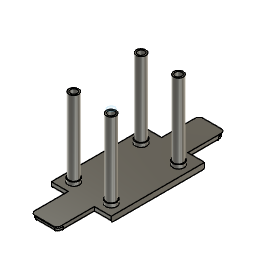
Micromouse_Gesamtaufbau_v8 (Autodesk Fusion 360 archive; units mm, degrees)
design "Mouse_Layout_MotorMount"
Autodesk Fusion 360 part; units mm, degrees
sketch "Skizze1" plane through (0, 0, 0) normal (0, 0, 1) x (1, 0, 0)
  line L0 (45, -30) -> (45, -50)
  line L1 (45, -50) -> (-45, -50)
  line L2 (-45, -50) -> (-45, -30)
  arc A0 (45, 0) -> (-45, 0) centre (0, 0) ccw
  line L3 (-45, 0) -> (-36, 0)
  line L4 (-36, 0) -> (-36, -30)
  line L5 (-36, -30) -> (-45, -30)
  line L6 (36, 0) -> (36, -30)
  line L7 (36, -30) -> (45, -30)
  line L8 (36, 0) -> (45, 0)
  dimension "d1" = 90
  dimension "d2" = 50
  dimension "d3" = 9
  dimension "d4" = 30
  dimension "d5" = 9
  dimension "d6" = 30
  constraint coincident A0.centre origin
  constraint vertical L0
  constraint horizontal L1
  constraint vertical L2
  constraint horizontal L3
  constraint vertical L4
  constraint horizontal L5
  constraint vertical L6
  constraint horizontal L7
  measures "d1" diameter of A0
  measures "d2" distance of A0.end L1.end
  measures "d3" distance of A0.end L3.end
  measures "d4" distance of A0.end L2.end
  measures "d5" distance of A0.start L6.start
  measures "d6" distance of A0.start L0.start
extrude "Extrusion1" add sketch "Skizze1" along normal blind 1.6 makes body 1
sketch "Skizze2" plane through (0, 0, 1.6) normal (0, 0, 1) x (-1, 0, 0)
  line L0 (-36, 30) -> (-36, 0)
  line L1 (-36, 0) -> (-45, 0)
  arc A0 (-45, 0) -> (45, 0) centre (0, 0) ccw
  line L2 (45, 0) -> (36, 0)
  line L3 (36, 0) -> (36, 30)
  line L4 (36, 30) -> (45, 30)
  line L5 (45, 30) -> (45, 50)
  line L6 (45, 50) -> (-45, 50)
  line L7 (-45, 50) -> (-45, 30)
  line L8 (-45, 30) -> (-36, 30)
  line L9 (36, 15) -> (36, 24)
  line L10 (36, 15) -> (36, 6)
  circle A1 centre (26, 24) radius 1.5
  circle A2 centre (16, 24) radius 1.5
  circle A3 centre (26, 6) radius 1.5
  circle A4 centre (16, 6) radius 1.5
  line L11 (36, 15) -> (36, 9)
  line L12 (36, 9) -> (11, 9)
  line L13 (11, 9) -> (11, 21)
  line L14 (11, 21) -> (36, 21)
  line L15 (36, 21) -> (36, 9)
  line L16 (36, 24) -> (36, 27)
  line L17 (36, 27) -> (4, 27)
  line L18 (4, 27) -> (4, 2)
  line L19 (4, 2) -> (36, 2)
  line L20 (36, 2) -> (36, 27)
  line L21 (-36, 27) -> (-4, 27)
  line L22 (-4, 27) -> (-4, 2)
  line L23 (-4, 2) -> (-36, 2)
  line L24 (-36, 2) -> (-36, 27)
  line L25 (-11, 21) -> (-36, 21)
  line L26 (-36, 21) -> (-11, 21)
  line L27 (-11, 21) -> (-11, 9)
  line L28 (-11, 9) -> (-36, 9)
  line L29 (-36, 9) -> (-36, 21)
  circle A5 centre (-16, 6) radius 1.5
  circle A6 centre (-26, 6) radius 1.5
  circle A7 centre (-16, 24) radius 1.5
  circle A8 centre (-26, 24) radius 1.5
  dimension "d10" = 9
  dimension "d11" = 9
  dimension "d12" = 10
  dimension "d13" = 10
  dimension "d14" = 10
  dimension "d15" = 10
  dimension "d16" = 3
  dimension "d17" = 3
  dimension "d18" = 3
  dimension "d19" = 3
  dimension "d20" = 6
  dimension "d21" = 25
  dimension "d22" = 12
  dimension "d23" = 3
  dimension "d24" = 32
  dimension "d25" = 25
  dimension "d30" = 32
  dimension "d31" = 25
  dimension "d32" = 25
  dimension "d33" = 12
  dimension "d35" = 10
  dimension "d37" = 10
  dimension "d38" = 3
  dimension "d39" = 3
  dimension "d40" = 3
  dimension "d41" = 3
  dimension "d42" = 10
  dimension "d43" = 10
  constraint midpoint L3 L9.start
  constraint horizontal L12
  constraint vertical L13
  constraint horizontal L14
  constraint vertical L15
  constraint coincident L3 L16.end
  constraint parallel L3 L16
  constraint horizontal L17
  constraint vertical L18
  constraint horizontal L19
  constraint vertical L20
  constraint coincident L0 L21.start
  constraint horizontal L21
  constraint vertical L22
  constraint horizontal L23
  constraint vertical L24
  constraint perpendicular L22 L25
  constraint horizontal L26
  constraint vertical L27
  constraint horizontal L28
  constraint vertical L29
  measures "d10" distance of L9.start L9.end
  measures "d11" distance of L9.start L10.end
  measures "d12" distance of L10.end A3.centre
  measures "d13" distance of A3.centre A4.centre
  measures "d14" distance of L9.end A1.centre
  measures "d15" distance of A1.centre A2.centre
  measures "d16" diameter of A1
  measures "d17" diameter of A2
  measures "d18" diameter of A3
  measures "d19" diameter of A4
  measures "d20" distance of L9.start L11.end
  measures "d21" distance of L11.end L12.end
  measures "d22" distance of L11.end L14.end
  measures "d23" distance of L9.end L16.end
  measures "d24" distance of L16.end L17.end
  measures "d25" distance of L16.end L19.end
  measures "d30" distance of L21.start L21.end
  measures "d31" distance of L21.start L23.end
  measures "d32" distance of L25.end L25.start
  measures "d33" distance of L25.end L28.end
  measures "d35" distance of A5.centre A6.centre
  measures "d37" distance of A7.centre A8.centre
  measures "d38" diameter of A5
  measures "d39" diameter of A6
  measures "d40" diameter of A7
  measures "d41" diameter of A8
  measures "d42" distance of L24 A6.centre
  measures "d43" distance of L24 A8.centre
extrude "Extrusion2" cut sketch "Skizze2" against normal blind 1.6 contours A1 | A2 | A3 | A4 bodies 1
mirror "Spiegeln1" about plane through (0, 0, 0) normal (1, 0, 0) of "Extrusion2"
extrude "Extrusion3" cut sketch "Skizze2" against normal blind 2 contours L0 L1 A0 L2 L3 L4 L5 L6 L7 L8 L17 L18 L19 L21 L22 L23 bodies 1 makes body 2 at (7.5869, -11.9483, 0)
extrude "Extrusion4" cut sketch "Skizze2" against normal blind 2 contours L0 L1 A0 L2 L3 L4 L5 L6 L7 L8 L17 L18 L19 L21 L22 L23 bodies 2 1
extrude "Extrusion5" cut sketch "Skizze2" against normal blind 2 contours L0 L21 L22 L23 L24 L25 L26 L27 L28 | L0 L24 L25 L26 L27 L28 L29 bodies 2
sketch "Skizze3" plane through (0, 0, 0) normal (0, 0, -1) x (1, 0, 0)
  line L0 (-36, 2) -> (-4, 2)
  line L1 (-4, 2) -> (-4, 27)
  line L2 (-4, 27) -> (-36, 27)
  line L3 (-36, 27) -> (-36, 2)
  circle A0 centre (-26, 24) radius 1.5
  circle A1 centre (-26, 6) radius 1.5
  circle A2 centre (-16, 24) radius 1.5
  circle A3 centre (-16, 6) radius 1.5
  line L4 (-29, 27) -> (-13, 27)
  line L5 (-13, 27) -> (-13, 2)
  line L6 (-13, 2) -> (-29, 2)
  line L7 (-29, 2) -> (-29, 27)
  circle A4 centre (-26, 24) radius 1.5
  circle A5 centre (-16, 24) radius 1.5
  circle A6 centre (-16, 6) radius 1.5
  circle A7 centre (-26, 6) radius 1.5
  constraint horizontal L4
  constraint vertical L5
  constraint horizontal L6
  constraint vertical L7
  constraint coincident L0 L5.end
  constraint coincident L2 L4.start
  constraint concentric A0 A4
  constraint concentric A2 A5
  constraint concentric A3 A6
  constraint concentric A1 A7
extrude "Extrusion6" add sketch "Skizze3" along normal blind 1.9 contours L0 L2 L4 L5 L6 L7 | A0 A4 | A1 A7 | A2 A5 | A3 A6 bodies 1 2
extrude "Extrusion7" cut sketch "Skizze2" against normal blind 1.6 contours L3 L9 L10 L12 L13 L14 L16 L17 L18 L19 L20 | L3 L9 L10 L11 L12 L13 L14 L15 L20 bodies 1
extrude "Extrusion8" add sketch "Skizze3" against normal blind 21.9 contours A0 A4 | A1 A7 | A2 A5 | A3 A6 bodies 1
sketch "Skizze4" plane through (0, -27, 0) normal (0, -1, 0) x (1, 0, 0)
  line L0 (-13, 0) -> (-29, 0)
  line L1 (-29, 0) -> (-29, -1.9)
  line L2 (-29, -1.9) -> (-13, -1.9)
  line L3 (-13, -1.9) -> (-13, 0)
  line L4 (-24.5, 0) -> (-17.5, 0)
  line L5 (-17.5, 0) -> (-17.5, -1.9)
  line L6 (-17.5, -1.9) -> (-24.5, -1.9)
  line L7 (-24.5, -1.9) -> (-24.5, 0)
  dimension "d56" = 7
  constraint horizontal L4
  constraint vertical L5
  constraint horizontal L6
  constraint vertical L7
  constraint coincident L2 L5.end
  constraint coincident L0 L4.start
  measures "d56" distance of L4.start L4.end
extrude "Extrusion9" add sketch "Skizze4" along normal blind 10 contours L0 L2 L4 L5 L6 L7 bodies 1
sketch "Skizze5" plane through (0, -2, 0) normal (0, 1, 0) x (-1, 0, 0)
  line L0 (29, 0) -> (13, 0)
  line L1 (13, 0) -> (13, -1.9)
  line L2 (13, -1.9) -> (29, -1.9)
  line L3 (29, -1.9) -> (29, 0)
  line L4 (17.5, 0) -> (24.5, 0)
  line L5 (24.5, 0) -> (24.5, -1.9)
  line L6 (24.5, -1.9) -> (17.5, -1.9)
  line L7 (17.5, -1.9) -> (17.5, 0)
  constraint horizontal L4
  constraint vertical L5
  constraint horizontal L6
  constraint vertical L7
  constraint coincident L2 L5.end
  constraint coincident L0 L4.start
extrude "Extrusion10" add sketch "Skizze5" along normal blind 10 contours L0 L2 L4 L5 L6 L7 bodies 1
fillet "Abrundung1" radius 3.5 2 edges at (-21, -37, -1.9) (-21, 8, -1.9) on bodies 1
fillet "Abrundung2" radius 1 14 edges at (-24.5, 1.4436, -1.9) (-24.5, 6.7106, -1.3875) (-17.5, 1.4436, -1.9) (-17.5, 6.7106, -1.3875) (-13, -14.5, -1.9) (-26.75, -2, -1.9) (-15.25, -2, -1.9) (-15.25, -27, -1.9) (-17.5, -30.4436, -1.9) (-17.5, -35.7106, -1.3875) (-24.5, -30.4436, -1.9) (-24.5, -35.7106, -1.3875) (-26.75, -27, -1.9) (-29, -14.5, -1.9) on bodies 1
sketch "Skizze6" plane through (0, 0, 21.9) normal (0, 0, 1) x (-1, 0, 0)
  circle A0 centre (26, 6) radius 1.5
  circle A1 centre (26, 6) radius 0.9
  circle A2 centre (16, 6) radius 0.9
  circle A3 centre (26, 24) radius 0.9
  circle A4 centre (16, 24) radius 0.9
  dimension "d65" = 1.8
  dimension "d66" = 1.8
  dimension "d67" = 1.8
  dimension "d68" = 1.8
  constraint concentric A0 A1
  measures "d65" diameter of A1
  measures "d66" diameter of A2
  measures "d67" diameter of A3
  measures "d68" diameter of A4
extrude "Extrusion11" cut sketch "Skizze6" against normal blind 12 contours A1 | A2 | A3 | A4 bodies 1
fillet "Abrundung3" radius 0.5 4 edges at (-27.3985, -6.5424, 21.9) (-17.3985, -6.5424, 21.9) (-17.3985, -24.5424, 21.9) (-27.3985, -24.5424, 21.9) on bodies 1
sketch "Skizze7" plane through (0, 0, 21.9) normal (0, 0, 1) x (-1, 0, 0)
  circle A0 centre (16, 24) radius 0.9
  circle A1 centre (16, 24) radius 1
  circle A2 centre (26, 6) radius 1.3
  circle A3 centre (16, 6) radius 1.3
  circle A4 centre (26, 24) radius 1.3
  circle A5 centre (16, 24) radius 1.3
  circle A6 centre (26, 6) radius 1.5
  circle A7 centre (16, 6) radius 1.5
  circle A8 centre (26, 24) radius 1.5
  circle A9 centre (16, 24) radius 1.5
  dimension "d73" = 2.6
  dimension "d74" = 2.6
  dimension "d75" = 2.6
  dimension "d76" = 3
  dimension "d77" = 3
  dimension "d78" = 3
  dimension "d79" = 3
  dimension "d82" = 2.6
  constraint concentric A0 A5
  constraint concentric A2 A6
  constraint concentric A3 A7
  constraint concentric A4 A8
  constraint concentric A5 A9
  measures "d73" diameter of A3
  measures "d74" diameter of A4
  measures "d75" diameter of A5
  measures "d76" diameter of A6
  measures "d77" diameter of A7
  measures "d78" diameter of A8
  measures "d79" diameter of A9
  measures "d82" diameter of A2
extrude "Extrusion12" cut sketch "Skizze7" against normal blind 21.9 contours A6 | A7 | A8 | A9 bodies 1
sketch "Skizze8" plane through (0, 0, -1.9) normal (0, 0, -1) x (1, 0, 0)
  line L0 (-18.5, 26) -> (-18.5, 33.8871)
  line L1 (-18.5, 33.8871) -> (-23.5, 33.8871)
  line L2 (-23.5, 33.8871) -> (-23.5, 26)
  line L3 (-23.5, 26) -> (-28, 26)
  line L4 (-28, 26) -> (-28, 3)
  line L5 (-28, 3) -> (-23.5, 3)
  line L6 (-23.5, 3) -> (-23.5, -4.8871)
  line L7 (-23.5, -4.8871) -> (-18.5, -4.8871)
  line L8 (-18.5, -4.8871) -> (-18.5, 3)
  line L9 (-18.5, 3) -> (-14, 3)
  line L10 (-14, 3) -> (-14, 26)
  line L11 (-14, 26) -> (-18.5, 26)
  line L12 (-13, 27) -> (-13, 2)
  line L13 (-29, 2) -> (-29, 27)
  line L14 (-13, 27) -> (-13, 37)
  line L15 (-13, 37) -> (-29, 37)
  line L16 (-29, 37) -> (-29, 27)
  line L17 (-13, 2) -> (-13, -8)
  line L18 (-13, -8) -> (-29, -8)
  line L19 (-29, -8) -> (-29, 2)
  constraint vertical L12
  constraint vertical L13
  constraint vertical L14
  constraint horizontal L15
  constraint vertical L16
  constraint vertical L17
  constraint horizontal L18
  constraint vertical L19
extrude "Extrusion13" cut sketch "Skizze8" against normal blind 1.4 contours L0 L1 L2 L3 L4 L5 L6 L7 L8 L9 L10 L11 | L12 L13 L14 L15 L16 L17 L18 L19 bodies 1
sketch "Skizze9" plane through (0, 0, 0) normal (0, 0, 1) x (-1, 0, 0)
  circle A0 centre (16, 6) radius 1.3
  circle A1 centre (26, 24) radius 1.3
  circle A2 centre (26, 6) radius 1.3
  circle A3 centre (16, 24) radius 1.3
  spline S0 degree 3 poles (17.5, 35.8081) (17.5, 35.9658) (17.5285, 36.153) (17.627, 36.4268) (17.7057, 36.566) (17.8787, 36.7656) (18.0032, 36.8615) (18.2336, 36.9678) (18.3773, 37) (18.5, 37) knots 1.603619 1.603619 1.603619 1.603619 1.650953 1.650953 1.690911 1.690911 1.730212 1.730212 1.767024 1.767024 1.767024 1.767024
  line L0 (17.5, 35.8081) -> (17.5, 27)
  line L1 (17.5, 27) -> (13, 27)
  line L2 (13, 27) -> (13, 2)
  line L3 (13, 2) -> (17.5, 2)
  line L4 (17.5, 2) -> (17.5, -6.8081)
  spline S1 degree 3 poles (18.5, -8) (18.3827, -8) (18.245, -7.9706) (18.0235, -7.8732) (17.9025, -7.7854) (17.7235, -7.593) (17.6383, -7.4507) (17.531, -7.1676) (17.5, -6.9726) (17.5, -6.8081) knots 1.060205 1.060205 1.060205 1.060205 1.095405 1.095405 1.132785 1.132785 1.174245 1.174245 1.223607 1.223607 1.223607 1.223607
  line L5 (18.5, -8) -> (23.5, -8)
  spline S2 degree 3 poles (24.5, -6.8081) (24.5, -6.9726) (24.469, -7.1676) (24.3617, -7.4507) (24.2765, -7.593) (24.0975, -7.7854) (23.9765, -7.8732) (23.755, -7.9706) (23.6173, -8) (23.5, -8) knots 1.603606 1.603606 1.603606 1.603606 1.652968 1.652968 1.694428 1.694428 1.731808 1.731808 1.767008 1.767008 1.767008 1.767008
  line L6 (24.5, -6.8081) -> (24.5, 2)
  line L7 (24.5, 2) -> (29, 2)
  line L8 (29, 2) -> (29, 27)
  line L9 (29, 27) -> (24.5, 27)
  line L10 (24.5, 27) -> (24.5, 35.8081)
  spline S3 degree 3 poles (23.5, 37) (23.6227, 37) (23.7664, 36.9678) (23.9968, 36.8615) (24.1213, 36.7656) (24.2943, 36.566) (24.373, 36.4268) (24.4715, 36.153) (24.5, 35.9658) (24.5, 35.8081) knots 1.060215 1.060215 1.060215 1.060215 1.097027 1.097027 1.136328 1.136328 1.176286 1.176286 1.22362 1.22362 1.22362 1.22362
  line L11 (23.5, 37) -> (18.5, 37)
  circle A4 centre (16, 6) radius 1.3
  circle A5 centre (16, 6) radius 1.5
  circle A6 centre (26, 6) radius 1.3
  circle A7 centre (26, 6) radius 1.5
  circle A8 centre (16, 24) radius 1.3
  circle A9 centre (16, 24) radius 1.5
  circle A10 centre (26, 24) radius 1.3
  circle A11 centre (26, 24) radius 1.5
  constraint concentric A0 A4
  constraint concentric A4 A5
  constraint concentric A2 A6
  constraint concentric A2 A7
  constraint concentric A3 A8
  constraint concentric A8 A9
  constraint concentric A1 A10
  constraint concentric A10 A11
extrude "Extrusion14" add sketch "Skizze9" along normal blind 1 contours A5 | A7 | A9 | A11 bodies 1
extrude "Extrusion15" add 1 faces at (-22.1667, -18.6667, -0.5) along direction (0, 0, -1) blind 1 on bodies 1 bodies 1
sketch "Skizze10" plane through (0, 0, 21.9) normal (0, 0, 1) x (-1, 0, 0)
  circle A0 centre (16, 24) radius 0.9
  circle A1 centre (16, 24) radius 1
sketch "Skizze11" plane through (0, 0, 0) normal (1, 0, 0) x (0, 1, 0)
  line L0 (-25, 21.9) -> (-25.5, 21.9)
  line L1 (-25.5, 21.9) -> (-25.5, 20.9)
  line L2 (-25.5, 20.9) -> (-4, 20.9)
  line L3 (-4, 20.9) -> (-4, 21.9)
  line L4 (-4, 21.9) -> (-25, 21.9)
  constraint horizontal L0
  constraint perpendicular L0 L1
  constraint perpendicular L1 L2
  constraint perpendicular L2 L3
  constraint perpendicular L1 L4
extrude "Extrusion16" cut sketch "Skizze11" against normal blind 32 bodies 1
fillet "Abrundung5" radius 0.5 14 edges at (-17.5, -31.1218, -1.5) (-17.7132, -36.1881, -1.5) (-21, -36.6871, -1.5) (-24.2868, -36.1881, -1.5) (-24.5, -31.1218, -1.5) (-24.5, 2.1218, -1.5) (-24.2859, 7.1906, -1.5) (-21, 7.6871, -1.5) (-17.7141, 7.1906, -1.5) (-17.5, 2.1218, -1.5) (-15.25, -27, -1.5) (-26.75, -27, -1.5) (-26.75, -2, -1.5) (-15.25, -2, -1.5) on bodies 1

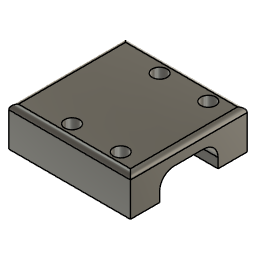
design "Mouse_Motor_Clamp_Upper"
Autodesk Fusion 360 part; units mm, degrees
sketch "Skizze1" plane through (0, 0, 0) normal (0, 0, 1) x (1, 0, 0)
  line L0 (45, -30) -> (45, -50)
  line L1 (45, -50) -> (-45, -50)
  line L2 (-45, -50) -> (-45, -30)
  arc A0 (45, 0) -> (-45, 0) centre (0, 0) ccw
  line L3 (-45, 0) -> (-36, 0)
  line L4 (-36, 0) -> (-36, -30)
  line L5 (-36, -30) -> (-45, -30)
  line L6 (36, 0) -> (36, -30)
  line L7 (36, -30) -> (45, -30)
  line L8 (36, 0) -> (45, 0)
  dimension "d1" = 90
  dimension "d2" = 50
  dimension "d3" = 9
  dimension "d4" = 30
  dimension "d5" = 9
  dimension "d6" = 30
  constraint coincident A0.centre origin
  constraint vertical L0
  constraint horizontal L1
  constraint vertical L2
  constraint horizontal L3
  constraint vertical L4
  constraint horizontal L5
  constraint vertical L6
  constraint horizontal L7
  measures "d1" diameter of A0
  measures "d2" distance of A0.end L1.end
  measures "d3" distance of A0.end L3.end
  measures "d4" distance of A0.end L2.end
  measures "d5" distance of A0.start L6.start
  measures "d6" distance of A0.start L0.start
extrude "Extrusion1" add sketch "Skizze1" along normal blind 1.6 makes body 1
sketch "Skizze2" plane through (0, 0, 1.6) normal (0, 0, 1) x (-1, 0, 0)
  line L0 (-36, 30) -> (-36, 0)
  line L1 (-36, 0) -> (-45, 0)
  arc A0 (-45, 0) -> (45, 0) centre (0, 0) ccw
  line L2 (45, 0) -> (36, 0)
  line L3 (36, 0) -> (36, 30)
  line L4 (36, 30) -> (45, 30)
  line L5 (45, 30) -> (45, 50)
  line L6 (45, 50) -> (-45, 50)
  line L7 (-45, 50) -> (-45, 30)
  line L8 (-45, 30) -> (-36, 30)
  line L9 (36, 15) -> (36, 24)
  line L10 (36, 15) -> (36, 6)
  circle A1 centre (26, 24) radius 1.525
  circle A2 centre (16, 24) radius 1.525
  circle A3 centre (26, 6) radius 1.525
  circle A4 centre (16, 6) radius 1.525
  line L11 (36, 15) -> (36, 9)
  line L12 (36, 9) -> (11, 9)
  line L13 (11, 9) -> (11, 21)
  line L14 (11, 21) -> (36, 21)
  line L15 (36, 21) -> (36, 9)
  line L16 (36, 24) -> (36, 27)
  line L17 (36, 27) -> (4, 27)
  line L18 (4, 27) -> (4, 2)
  line L19 (4, 2) -> (36, 2)
  line L20 (36, 2) -> (36, 27)
  line L21 (-36, 27) -> (-4, 27)
  line L22 (-4, 27) -> (-4, 2)
  line L23 (-4, 2) -> (-36, 2)
  line L24 (-36, 2) -> (-36, 27)
  line L25 (-11, 21) -> (-36, 21)
  line L26 (-36, 21) -> (-11, 21)
  line L27 (-11, 21) -> (-11, 9)
  line L28 (-11, 9) -> (-36, 9)
  line L29 (-36, 9) -> (-36, 21)
  circle A5 centre (-16, 6) radius 1.5
  circle A6 centre (-26, 6) radius 1.5
  circle A7 centre (-16, 24) radius 1.5
  circle A8 centre (-26, 24) radius 1.5
  dimension "d10" = 9
  dimension "d11" = 9
  dimension "d12" = 10
  dimension "d13" = 10
  dimension "d14" = 10
  dimension "d15" = 10
  dimension "d16" = 3.05
  dimension "d17" = 3.05
  dimension "d18" = 3.05
  dimension "d19" = 3.05
  dimension "d20" = 6
  dimension "d21" = 25
  dimension "d22" = 12
  dimension "d23" = 3
  dimension "d24" = 32
  dimension "d25" = 25
  dimension "d30" = 32
  dimension "d31" = 25
  dimension "d32" = 25
  dimension "d33" = 12
  dimension "d35" = 10
  dimension "d37" = 10
  dimension "d38" = 3
  dimension "d39" = 3
  dimension "d40" = 3
  dimension "d41" = 3
  dimension "d42" = 10
  dimension "d43" = 10
  constraint midpoint L3 L9.start
  constraint horizontal L12
  constraint vertical L13
  constraint horizontal L14
  constraint vertical L15
  constraint coincident L3 L16.end
  constraint parallel L3 L16
  constraint horizontal L17
  constraint vertical L18
  constraint horizontal L19
  constraint vertical L20
  constraint coincident L0 L21.start
  constraint horizontal L21
  constraint vertical L22
  constraint horizontal L23
  constraint vertical L24
  constraint perpendicular L22 L25
  constraint horizontal L26
  constraint vertical L27
  constraint horizontal L28
  constraint vertical L29
  measures "d10" distance of L9.start L9.end
  measures "d11" distance of L9.start L10.end
  measures "d12" distance of L10.end A3.centre
  measures "d13" distance of A3.centre A4.centre
  measures "d14" distance of L9.end A1.centre
  measures "d15" distance of A1.centre A2.centre
  measures "d16" diameter of A1
  measures "d17" diameter of A2
  measures "d18" diameter of A3
  measures "d19" diameter of A4
  measures "d20" distance of L9.start L11.end
  measures "d21" distance of L11.end L12.end
  measures "d22" distance of L11.end L14.end
  measures "d23" distance of L9.end L16.end
  measures "d24" distance of L16.end L17.end
  measures "d25" distance of L16.end L19.end
  measures "d30" distance of L21.start L21.end
  measures "d31" distance of L21.start L23.end
  measures "d32" distance of L25.end L25.start
  measures "d33" distance of L25.end L28.end
  measures "d35" distance of A5.centre A6.centre
  measures "d37" distance of A7.centre A8.centre
  measures "d38" diameter of A5
  measures "d39" diameter of A6
  measures "d40" diameter of A7
  measures "d41" diameter of A8
  measures "d42" distance of L24 A6.centre
  measures "d43" distance of L24 A8.centre
extrude "Extrusion2" cut sketch "Skizze2" against normal blind 1.6 contours A1 | A2 | A3 | A4 bodies 1
mirror "Spiegeln1" about plane through (0, 0, 0) normal (1, 0, 0) of "Extrusion2"
extrude "Extrusion3" cut sketch "Skizze2" against normal blind 2 contours L0 L1 A0 L2 L3 L4 L5 L6 L7 L8 L17 L18 L19 L21 L22 L23 bodies 1 makes body 2 at (7.58, -11.953, 0)
extrude "Extrusion12" cut sketch "Skizze2" against normal blind 2 contours L0 L21 L22 L23 L24 L25 L26 L27 L28 | L0 L24 L25 L26 L27 L28 L29 | L3 L9 L10 L12 L13 L14 L16 L17 L18 L19 L20 | L3 L9 L10 L11 L12 L13 L14 L15 L20 bodies 1 2
extrude "Extrusion13" add sketch "Skizze2" along normal blind 7.4 contours L3 L9 L10 L12 L13 L14 L16 L17 L18 L19 L20 | L3 L9 L10 L11 L12 L13 L14 L15 L20 bodies 1 2
extrude "Extrusion14" add 1 faces at (-7.58, -11.953, 9) along direction (0, 0, 1) blind 5 on bodies 1 bodies 1
extrude "Extrusion15" cut sketch "Skizze2" along normal blind 5 contours L3 L9 L10 L11 L12 L13 L14 L15 L20 bodies 1
sketch "Skizze7" plane through (0, 0, 1.6) normal (0, 0, 1) x (-1, 0, 0)
  line L0 (11, 27) -> (4, 27)
  line L1 (4, 27) -> (4, 2)
  line L2 (4, 2) -> (11, 2)
  line L3 (11, 2) -> (11, 27)
  constraint horizontal L0
  constraint vertical L1
  constraint horizontal L2
  constraint vertical L3
extrude "Extrusion16" cut sketch "Skizze7" along normal blind 13 bodies 1
fillet "Abrundung4" radius 3 2 edges at (-23.5, -21, 6.6) (-23.5, -9, 6.6) on bodies 1
sketch "Skizze8" plane through (0, 0, 1.6) normal (0, 0, 1) x (-1, 0, 0)
  line L0 (26, 21) -> (26, 9)
  line L1 (26, 21) -> (36, 21)
  line L2 (36, 21) -> (36, 9)
  line L3 (36, 9) -> (26, 9)
  constraint vertical L0
  constraint horizontal L1
  constraint vertical L2
  constraint horizontal L3
extrude "Extrusion17" cut sketch "Skizze8" along normal blind 5 bodies 1
extrude "Extrusion18" cut 1 faces at (-33.0867, -11.953, 14) along direction (0, 0, -1) blind 4.4 on bodies 1 bodies 1
sketch "Skizze9" plane through (0, 0, 9.6) normal (0, 0, 1) x (-1, 0, 0)
  line L0 (11, 27) -> (11, 2)
  line L1 (11, 2) -> (36, 2)
  line L2 (36, 2) -> (36, 27)
  line L3 (36, 27) -> (11, 27)
  circle A0 centre (26, 24) radius 1.525
  circle A1 centre (16, 24) radius 1.525
  circle A2 centre (16, 6) radius 1.525
  circle A3 centre (26, 6) radius 1.525
  line L4 (11, 2) -> (36, 2)
  line L5 (36, 2) -> (36, 3)
  line L6 (36, 3) -> (11, 3)
  line L7 (11, 3) -> (11, 2)
  dimension "d91" = 25
  constraint horizontal L4
  constraint vertical L5
  constraint horizontal L6
  constraint vertical L7
  constraint coincident L0.end L1.start
  measures "d91" distance of L0.end L1.end
extrude "Extrusion19" cut sketch "Skizze9" against normal blind 20 contours L0 L1 L2 L4 L5 L6 L7 bodies 1
fillet "Abrundung6" radius 1 4 edges at (-36, -15, 9.6) (-23.5, -3, 9.6) (-11, -15, 9.6) (-23.5, -27, 9.6) on bodies 1

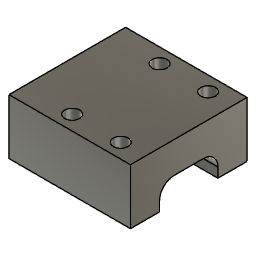
design "Mouse_Motor_Clamp_Lower"
Autodesk Fusion 360 part; units mm, degrees
sketch "Skizze1" plane through (0, 0, 0) normal (0, 0, 1) x (1, 0, 0)
  line L0 (45, -30) -> (45, -50)
  line L1 (45, -50) -> (-45, -50)
  line L2 (-45, -50) -> (-45, -30)
  arc A0 (45, 0) -> (-45, 0) centre (0, 0) ccw
  line L3 (-45, 0) -> (-36, 0)
  line L4 (-36, 0) -> (-36, -30)
  line L5 (-36, -30) -> (-45, -30)
  line L6 (36, 0) -> (36, -30)
  line L7 (36, -30) -> (45, -30)
  line L8 (36, 0) -> (45, 0)
  dimension "d1" = 90
  dimension "d2" = 50
  dimension "d3" = 9
  dimension "d4" = 30
  dimension "d5" = 9
  dimension "d6" = 30
  constraint coincident A0.centre origin
  constraint vertical L0
  constraint horizontal L1
  constraint vertical L2
  constraint horizontal L3
  constraint vertical L4
  constraint horizontal L5
  constraint vertical L6
  constraint horizontal L7
  measures "d1" diameter of A0
  measures "d2" distance of A0.end L1.end
  measures "d3" distance of A0.end L3.end
  measures "d4" distance of A0.end L2.end
  measures "d5" distance of A0.start L6.start
  measures "d6" distance of A0.start L0.start
extrude "Extrusion1" add sketch "Skizze1" along normal blind 1.6 makes body 1
sketch "Skizze2" plane through (0, 0, 1.6) normal (0, 0, 1) x (-1, 0, 0)
  line L0 (-36, 30) -> (-36, 0)
  line L1 (-36, 0) -> (-45, 0)
  arc A0 (-45, 0) -> (45, 0) centre (0, 0) ccw
  line L2 (45, 0) -> (36, 0)
  line L3 (36, 0) -> (36, 30)
  line L4 (36, 30) -> (45, 30)
  line L5 (45, 30) -> (45, 50)
  line L6 (45, 50) -> (-45, 50)
  line L7 (-45, 50) -> (-45, 30)
  line L8 (-45, 30) -> (-36, 30)
  line L9 (36, 15) -> (36, 24)
  line L10 (36, 15) -> (36, 6)
  circle A1 centre (26, 24) radius 1.525
  circle A2 centre (16, 24) radius 1.525
  circle A3 centre (26, 6) radius 1.525
  circle A4 centre (16, 6) radius 1.525
  line L11 (36, 15) -> (36, 9)
  line L12 (36, 9) -> (11, 9)
  line L13 (11, 9) -> (11, 21)
  line L14 (11, 21) -> (36, 21)
  line L15 (36, 21) -> (36, 9)
  line L16 (36, 24) -> (36, 27)
  line L17 (36, 27) -> (4, 27)
  line L18 (4, 27) -> (4, 2)
  line L19 (4, 2) -> (36, 2)
  line L20 (36, 2) -> (36, 27)
  line L21 (-36, 27) -> (-4, 27)
  line L22 (-4, 27) -> (-4, 2)
  line L23 (-4, 2) -> (-36, 2)
  line L24 (-36, 2) -> (-36, 27)
  line L25 (-11, 21) -> (-36, 21)
  line L26 (-36, 21) -> (-11, 21)
  line L27 (-11, 21) -> (-11, 9)
  line L28 (-11, 9) -> (-36, 9)
  line L29 (-36, 9) -> (-36, 21)
  circle A5 centre (-16, 6) radius 1.5
  circle A6 centre (-26, 6) radius 1.5
  circle A7 centre (-16, 24) radius 1.5
  circle A8 centre (-26, 24) radius 1.5
  dimension "d10" = 9
  dimension "d11" = 9
  dimension "d12" = 10
  dimension "d13" = 10
  dimension "d14" = 10
  dimension "d15" = 10
  dimension "d16" = 3.05
  dimension "d17" = 3.05
  dimension "d18" = 3.05
  dimension "d19" = 3.05
  dimension "d20" = 6
  dimension "d21" = 25
  dimension "d22" = 12
  dimension "d23" = 3
  dimension "d24" = 32
  dimension "d25" = 25
  dimension "d30" = 32
  dimension "d31" = 25
  dimension "d32" = 25
  dimension "d33" = 12
  dimension "d35" = 10
  dimension "d37" = 10
  dimension "d38" = 3
  dimension "d39" = 3
  dimension "d40" = 3
  dimension "d41" = 3
  dimension "d42" = 10
  dimension "d43" = 10
  constraint midpoint L3 L9.start
  constraint horizontal L12
  constraint vertical L13
  constraint horizontal L14
  constraint vertical L15
  constraint coincident L3 L16.end
  constraint parallel L3 L16
  constraint horizontal L17
  constraint vertical L18
  constraint horizontal L19
  constraint vertical L20
  constraint coincident L0 L21.start
  constraint horizontal L21
  constraint vertical L22
  constraint horizontal L23
  constraint vertical L24
  constraint perpendicular L22 L25
  constraint horizontal L26
  constraint vertical L27
  constraint horizontal L28
  constraint vertical L29
  measures "d10" distance of L9.start L9.end
  measures "d11" distance of L9.start L10.end
  measures "d12" distance of L10.end A3.centre
  measures "d13" distance of A3.centre A4.centre
  measures "d14" distance of L9.end A1.centre
  measures "d15" distance of A1.centre A2.centre
  measures "d16" diameter of A1
  measures "d17" diameter of A2
  measures "d18" diameter of A3
  measures "d19" diameter of A4
  measures "d20" distance of L9.start L11.end
  measures "d21" distance of L11.end L12.end
  measures "d22" distance of L11.end L14.end
  measures "d23" distance of L9.end L16.end
  measures "d24" distance of L16.end L17.end
  measures "d25" distance of L16.end L19.end
  measures "d30" distance of L21.start L21.end
  measures "d31" distance of L21.start L23.end
  measures "d32" distance of L25.end L25.start
  measures "d33" distance of L25.end L28.end
  measures "d35" distance of A5.centre A6.centre
  measures "d37" distance of A7.centre A8.centre
  measures "d38" diameter of A5
  measures "d39" diameter of A6
  measures "d40" diameter of A7
  measures "d41" diameter of A8
  measures "d42" distance of L24 A6.centre
  measures "d43" distance of L24 A8.centre
extrude "Extrusion2" cut sketch "Skizze2" against normal blind 1.6 contours A1 | A2 | A3 | A4 bodies 1
mirror "Spiegeln1" about plane through (0, 0, 0) normal (1, 0, 0) of "Extrusion2"
extrude "Extrusion3" cut sketch "Skizze2" against normal blind 2 contours L0 L1 A0 L2 L3 L4 L5 L6 L7 L8 L17 L18 L19 L21 L22 L23 bodies 1 makes body 2 at (7.58, -11.953, 0)
extrude "Extrusion12" cut sketch "Skizze2" against normal blind 2 contours L0 L21 L22 L23 L24 L25 L26 L27 L28 | L0 L24 L25 L26 L27 L28 L29 | L3 L9 L10 L12 L13 L14 L16 L17 L18 L19 L20 | L3 L9 L10 L11 L12 L13 L14 L15 L20 bodies 1 2
extrude "Extrusion13" add sketch "Skizze2" along normal blind 7.4 contours L3 L9 L10 L12 L13 L14 L16 L17 L18 L19 L20 | L3 L9 L10 L11 L12 L13 L14 L15 L20 bodies 1 2
extrude "Extrusion14" add 1 faces at (-7.58, -11.953, 9) along direction (0, 0, 1) blind 5 on bodies 1 bodies 1
extrude "Extrusion15" cut sketch "Skizze2" along normal blind 5 contours L3 L9 L10 L11 L12 L13 L14 L15 L20 bodies 1
sketch "Skizze7" plane through (0, 0, 1.6) normal (0, 0, 1) x (-1, 0, 0)
  line L0 (11, 27) -> (4, 27)
  line L1 (4, 27) -> (4, 2)
  line L2 (4, 2) -> (11, 2)
  line L3 (11, 2) -> (11, 27)
  constraint horizontal L0
  constraint vertical L1
  constraint horizontal L2
  constraint vertical L3
extrude "Extrusion16" cut sketch "Skizze7" along normal blind 13 bodies 1
fillet "Abrundung4" radius 3 2 edges at (-23.5, -21, 6.6) (-23.5, -9, 6.6) on bodies 1
sketch "Skizze8" plane through (0, 0, 1.6) normal (0, 0, 1) x (-1, 0, 0)
  line L0 (26, 21) -> (26, 9)
  line L1 (26, 21) -> (36, 21)
  line L2 (36, 21) -> (36, 9)
  line L3 (36, 9) -> (26, 9)
  constraint vertical L0
  constraint horizontal L1
  constraint vertical L2
  constraint horizontal L3
extrude "Extrusion17" cut sketch "Skizze8" along normal blind 5 bodies 1
sketch "Skizze9" plane through (0, 0, 14) normal (0, 0, 1) x (-1, 0, 0)
  line L0 (11, 27) -> (11, 2)
  line L1 (11, 2) -> (36, 2)
  line L2 (36, 2) -> (36, 27)
  line L3 (36, 27) -> (11, 27)
  circle A0 centre (26, 24) radius 1.525
  circle A1 centre (16, 24) radius 1.525
  circle A2 centre (16, 6) radius 1.525
  circle A3 centre (26, 6) radius 1.525
  line L4 (36, 2) -> (11, 2)
  line L5 (11, 2) -> (11, 3)
  line L6 (11, 3) -> (36, 3)
  line L7 (36, 3) -> (36, 2)
  constraint horizontal L4
  constraint vertical L5
  constraint horizontal L6
  constraint vertical L7
  constraint coincident L0 L5.end
  constraint coincident L1.end L2.start
extrude "Extrusion18" cut sketch "Skizze9" against normal blind 20 contours L0 L1 L2 L4 L5 L6 L7 bodies 1
extrude "Extrusion19" cut 1 faces at (-33.0393, -17.6542, 14) along direction (0, 0, -1) blind 1 on bodies 1 bodies 1
